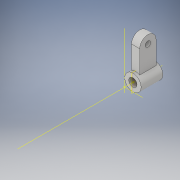
# Autodesk Inventor part: 7a
Saved by Autodesk Inventor 2018 (Build 220112000, 112)
## iProperties
Created: 2018-10-23
Part Number: 7a
Material: Generic
Document SubType Name: Modeling
Designer: Jerry
Density: 1 g/cm^3
Appearance: Default
Author: Jerry
Autodesk Inventor part; units mm, degrees
ref_plane "XZ Plane" through (0, 0, 0) normal (0, 1, 0) x (-1, 0, 0)
ref_plane "XY Plane" through (0, 0, 0) normal (0, 0, 1) x (1, 0, 0)
sketch "Sketch1" plane through (0, 0, 0) normal (0, 0, 1) x (1, 0, 0)
  circle A0 centre (0.75, 0.75) radius 0.75
  circle A1 centre (0.75, 0.75) radius 0.375
  line L0 (0.3443, 1.3808) -> (1.8045, 1.3808) construction
  point P0 (0, 0)
  dimension "d0" = 1.5
  dimension "d1" = 0.75
  constraints: 2 coincident, 2 end point, 1 centre point, 1 horizontal, 3 other
  measures "d1" diameter of A1
extrude "Extrusion1" add sketch "Sketch1" against normal blind 2
ref_plane "Work Plane1" through (0.75, 0.75, 0) normal (1, 0, 0) x (0, 1, 0)
sketch "Sketch2" plane through (0.75, 0.75, 0) normal (1, 0, 0) x (0, 1, 0)
  line L0 (-0.75, 0) -> (0.75, 0) projected
  line L1 (0, 0) -> (0, -3.3521)
  arc A0 (2.75, -1.75) -> (2.75, -0.25) centre (2.75, -1) ccw
  line L2 (2.75, -1) -> (2.75, -0.25) construction
  line L3 (2.75, -1) -> (2.75, -1.75) construction
  line L4 (2.75, -0.25) -> (0.404, -0.25)
  line L5 (2.75, -0.25) -> (5.096, -0.25) construction
  line L6 (0.404, -0.25) -> (0.404, -1.75)
  line L7 (0.404, -1.75) -> (2.75, -1.75)
  circle A1 centre (2.75, -1) radius 0.25
  dimension "d5" = 1
  dimension "d6" = 2.75
  dimension "d7" = 0.75
  dimension "d8" = 180
  dimension "d9" = 180
  dimension "d10" = 0.5
  constraints: 14 end point, 2 centre point, 2 coincident, 2 perpendicular, 2 point on circle, 1 collinear, 1 horizontal, 1 midpoint, 1 vertical
  measures "d5" distance from line of L0 point (2.75, -1)
  measures "d6" distance from line of L1 point (2.75, -1)
  measures "d7" radius of A0
  measures "d8" angle of L3 L2
  measures "d9" angle of L4 L5
  measures "d10" diameter of A1
extrude "Extrusion2" add sketch "Sketch2" along normal mid plane 0.75
body "Solid1"
